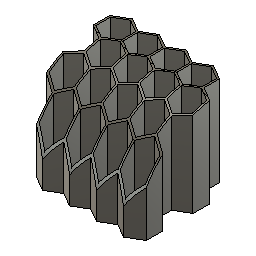
hexagon-03 (Autodesk Fusion 360 design; units mm, degrees)
Autodesk Fusion 360 part; units mm, degrees
sketch "Sketch1" plane through (0, 0, 0) normal (0, 1, 0) x (1, 0, 0)
  line L0 (16, 9.2376) -> (0, 18.4752)
  line L1 (0, 18.4752) -> (-16, 9.2376)
  line L2 (-16, 9.2376) -> (-16, -9.2376)
  line L3 (-16, -9.2376) -> (0, -18.4752)
  line L4 (0, -18.4752) -> (16, -9.2376)
  line L5 (16, -9.2376) -> (16, 9.2376)
  line L6 (46, 9.2376) -> (30, 18.4752)
  line L7 (30, 18.4752) -> (14, 9.2376)
  line L8 (14, 9.2376) -> (14, -9.2376)
  line L9 (14, -9.2376) -> (30, -18.4752)
  line L10 (30, -18.4752) -> (46, -9.2376)
  line L11 (46, -9.2376) -> (46, 9.2376)
  line L12 (14, 8.0829) -> (0, 16.1658)
  line L13 (0, 16.1658) -> (-14, 8.0829)
  line L14 (-14, 8.0829) -> (-14, -8.0829)
  line L15 (-14, -8.0829) -> (0, -16.1658)
  line L16 (0, -16.1658) -> (14, -8.0829)
  line L17 (14, -8.0829) -> (14, 8.0829)
  line L18 (44, 8.0829) -> (30, 16.1658)
  line L19 (30, 16.1658) -> (16, 8.0829)
  line L20 (16, 8.0829) -> (16, -8.0829)
  line L21 (16, -8.0829) -> (30, -16.1658)
  line L22 (30, -16.1658) -> (44, -8.0829)
  line L23 (44, -8.0829) -> (44, 8.0829)
  line L24 (15, -9.8342) -> (1, -17.9171)
  line L25 (59, -17.9171) -> (45, -9.8342)
  line L26 (15, -42.1658) -> (29, -34.0829)
  line L27 (29, -16.7624) -> (29, -35.2376)
  line L28 (-1, -16.7624) -> (-1, -35.2376)
  line L29 (29, -35.2376) -> (45, -44.4752)
  line L30 (29, -17.9171) -> (15, -9.8342)
  line L31 (61, -16.7624) -> (45, -7.5248)
  line L32 (45, -42.1658) -> (59, -34.0829)
  line L33 (59, -34.0829) -> (59, -17.9171)
  line L34 (61, -35.2376) -> (61, -16.7624)
  line L35 (45, -9.8342) -> (31, -17.9171)
  line L36 (31, -34.0829) -> (45, -42.1658)
  line L37 (15, -7.5248) -> (-1, -16.7624)
  line L38 (45, -7.5248) -> (29, -16.7624)
  line L39 (-1, -35.2376) -> (15, -44.4752)
  line L40 (45, -44.4752) -> (61, -35.2376)
  line L41 (1, -17.9171) -> (1, -34.0829)
  line L42 (31, -17.9171) -> (31, -34.0829)
  line L43 (31, -16.7624) -> (15, -7.5248)
  line L44 (15, -44.4752) -> (31, -35.2376)
  line L45 (29, -34.0829) -> (29, -17.9171)
  line L46 (1, -34.0829) -> (15, -42.1658)
  line L47 (31, -35.2376) -> (31, -16.7624)
  line L48 (89, -34.0829) -> (89, -17.9171)
  line L49 (60, -18.4752) -> (76, -9.2376)
  line L50 (76, 9.2376) -> (60, 18.4752)
  line L51 (59, -35.2376) -> (75, -44.4752)
  line L52 (75, -9.8342) -> (61, -17.9171)
  line L53 (75, -44.4752) -> (91, -35.2376)
  line L54 (75, -42.1658) -> (89, -34.0829)
  line L55 (119, -34.0829) -> (119, -17.9171)
  line L56 (121, -16.7624) -> (105, -7.5248)
  line L57 (90, -16.1658) -> (104, -8.0829)
  line L58 (105, -9.8342) -> (91, -17.9171)
  line L59 (60, 16.1658) -> (46, 8.0829)
  line L60 (44, -9.2376) -> (60, -18.4752)
  line L61 (74, -8.0829) -> (74, 8.0829)
  line L62 (74, -9.2376) -> (90, -18.4752)
  line L63 (105, -44.4752) -> (121, -35.2376)
  line L64 (74, 9.2376) -> (74, -9.2376)
  line L65 (46, 8.0829) -> (46, -8.0829)
  line L66 (59, -16.7624) -> (59, -35.2376)
  line L67 (90, 18.4752) -> (74, 9.2376)
  line L68 (76, 8.0829) -> (76, -8.0829)
  line L69 (91, -34.0829) -> (105, -42.1658)
  line L70 (89, -17.9171) -> (75, -9.8342)
  line L71 (105, -7.5248) -> (89, -16.7624)
  line L72 (119, -17.9171) -> (105, -9.8342)
  line L73 (104, 8.0829) -> (90, 16.1658)
  line L74 (60, 18.4752) -> (44, 9.2376)
  line L75 (90, 16.1658) -> (76, 8.0829)
  line L76 (90, -18.4752) -> (106, -9.2376)
  line L77 (76, -9.2376) -> (76, 9.2376)
  line L78 (106, -9.2376) -> (106, 9.2376)
  line L79 (106, 9.2376) -> (90, 18.4752)
  line L80 (74, 8.0829) -> (60, 16.1658)
  line L81 (89, -16.7624) -> (89, -35.2376)
  line L82 (61, -17.9171) -> (61, -34.0829)
  line L83 (105, -42.1658) -> (119, -34.0829)
  line L84 (91, -16.7624) -> (75, -7.5248)
  line L85 (91, -17.9171) -> (91, -34.0829)
  line L86 (91, -35.2376) -> (91, -16.7624)
  line L87 (75, -7.5248) -> (59, -16.7624)
  line L88 (121, -35.2376) -> (121, -16.7624)
  line L89 (61, -34.0829) -> (75, -42.1658)
  line L90 (76, -8.0829) -> (90, -16.1658)
  line L91 (89, -35.2376) -> (105, -44.4752)
  line L92 (46, -8.0829) -> (60, -16.1658)
  line L93 (104, -8.0829) -> (104, 8.0829)
  line L94 (44, 9.2376) -> (44, -9.2376)
  line L95 (60, -16.1658) -> (74, -8.0829)
  line L96 (16, 9.2376) -> (0, 18.4752)
  line L97 (0, -18.4752) -> (16, -9.2376)
  line L98 (0, -16.1658) -> (14, -8.0829)
  line L99 (104, -8.0829) -> (104, 8.0829)
  line L100 (90, -18.4752) -> (106, -9.2376)
  line L101 (44, 9.2376) -> (44, -9.2376)
  line L102 (-16, -9.2376) -> (0, -18.4752)
  line L103 (60, -18.4752) -> (76, -9.2376)
  line L104 (-14, 8.0829) -> (-14, -8.0829)
  line L105 (0, 16.1658) -> (-14, 8.0829)
  line L106 (90, 18.4752) -> (74, 9.2376)
  line L107 (60, 18.4752) -> (44, 9.2376)
  line L108 (76, -8.0829) -> (90, -16.1658)
  line L109 (-14, -8.0829) -> (0, -16.1658)
  line L110 (90, -16.1658) -> (104, -8.0829)
  line L111 (-1, -16.7624) -> (-1, -35.2376)
  line L112 (0, 18.4752) -> (-16, 9.2376)
  line L113 (60, -16.1658) -> (74, -8.0829)
  line L114 (1, -17.9171) -> (1, -34.0829)
  line L115 (46, -9.2376) -> (46, 9.2376)
  line L116 (44, -8.0829) -> (44, 8.0829)
  line L117 (45, -9.8342) -> (31, -17.9171)
  line L118 (30, 18.4752) -> (14, 9.2376)
  line L119 (30, -16.1658) -> (44, -8.0829)
  line L120 (59, -34.0829) -> (59, -17.9171)
  line L121 (45, -42.1658) -> (59, -34.0829)
  line L122 (89, -35.2376) -> (105, -44.4752)
  line L123 (59, -17.9171) -> (45, -9.8342)
  line L124 (31, -35.2376) -> (31, -16.7624)
  line L125 (15, -42.1658) -> (29, -34.0829)
  line L126 (14, -8.0829) -> (14, 8.0829)
  line L127 (61, -35.2376) -> (61, -16.7624)
  line L128 (31, -16.7624) -> (15, -7.5248)
  line L129 (30, 16.1658) -> (16, 8.0829)
  line L130 (61, -16.7624) -> (45, -7.5248)
  line L131 (16, -8.0829) -> (30, -16.1658)
  line L132 (15, -44.4752) -> (31, -35.2376)
  line L133 (44, 8.0829) -> (30, 16.1658)
  line L134 (61, -17.9171) -> (61, -34.0829)
  line L135 (45, -44.4752) -> (61, -35.2376)
  line L136 (60, 16.1658) -> (46, 8.0829)
  line L137 (16, -9.2376) -> (16, 9.2376)
  line L138 (14, 9.2376) -> (14, -9.2376)
  line L139 (45, -7.5248) -> (29, -16.7624)
  line L140 (29, -16.7624) -> (29, -35.2376)
  line L141 (30, -18.4752) -> (46, -9.2376)
  line L142 (14, -9.2376) -> (30, -18.4752)
  line L143 (14, 8.0829) -> (0, 16.1658)
  line L144 (1, -34.0829) -> (15, -42.1658)
  line L145 (15, -7.5248) -> (-1, -16.7624)
  line L146 (-1, -35.2376) -> (15, -44.4752)
  line L147 (121, -35.2376) -> (121, -16.7624)
  line L148 (31, -17.9171) -> (31, -34.0829)
  line L149 (105, -42.1658) -> (119, -34.0829)
  line L150 (91, -35.2376) -> (91, -16.7624)
  line L151 (119, -34.0829) -> (119, -17.9171)
  line L152 (91, -34.0829) -> (105, -42.1658)
  line L153 (59, -16.7624) -> (59, -35.2376)
  line L154 (31, -34.0829) -> (45, -42.1658)
  line L155 (29, -34.0829) -> (29, -17.9171)
  line L156 (29, -35.2376) -> (45, -44.4752)
  line L157 (75, -44.4752) -> (91, -35.2376)
  line L158 (89, -34.0829) -> (89, -17.9171)
  line L159 (75, -42.1658) -> (89, -34.0829)
  line L160 (59, -35.2376) -> (75, -44.4752)
  line L161 (16, 8.0829) -> (16, -8.0829)
  line L162 (29, -17.9171) -> (15, -9.8342)
  line L163 (89, -16.7624) -> (89, -35.2376)
  line L164 (105, -44.4752) -> (121, -35.2376)
  line L165 (91, -17.9171) -> (91, -34.0829)
  line L166 (61, -34.0829) -> (75, -42.1658)
  line L167 (106, 9.2376) -> (90, 18.4752)
  line L168 (15, -9.8342) -> (1, -17.9171)
  line L169 (-16, 9.2376) -> (-16, -9.2376)
  line L170 (74, -8.0829) -> (74, 8.0829)
  line L171 (90, 16.1658) -> (76, 8.0829)
  line L172 (76, 8.0829) -> (76, -8.0829)
  line L173 (75, -9.8342) -> (61, -17.9171)
  line L174 (121, -16.7624) -> (105, -7.5248)
  line L175 (106, -9.2376) -> (106, 9.2376)
  line L176 (76, 9.2376) -> (60, 18.4752)
  line L177 (91, -16.7624) -> (75, -7.5248)
  line L178 (105, -9.8342) -> (91, -17.9171)
  line L179 (46, 8.0829) -> (46, -8.0829)
  line L180 (105, -7.5248) -> (89, -16.7624)
  line L181 (46, 9.2376) -> (30, 18.4752)
  line L182 (89, -17.9171) -> (75, -9.8342)
  line L183 (46, -8.0829) -> (60, -16.1658)
  line L184 (104, 8.0829) -> (90, 16.1658)
  line L185 (76, -9.2376) -> (76, 9.2376)
  line L186 (119, -17.9171) -> (105, -9.8342)
  line L187 (74, 8.0829) -> (60, 16.1658)
  line L188 (74, -9.2376) -> (90, -18.4752)
  line L189 (44, -9.2376) -> (60, -18.4752)
  line L190 (75, -7.5248) -> (59, -16.7624)
  line L191 (74, 9.2376) -> (74, -9.2376)
  line L192 (15, -59.5248) -> (-1, -68.7624)
  line L193 (59, -68.7624) -> (59, -87.2376)
  line L194 (91, -69.9171) -> (91, -86.0829)
  line L195 (105, -94.1658) -> (119, -86.0829)
  line L196 (31, -87.2376) -> (31, -68.7624)
  line L197 (31, -69.9171) -> (31, -86.0829)
  line L198 (15, -96.4752) -> (31, -87.2376)
  line L199 (121, -87.2376) -> (121, -68.7624)
  line L200 (45, -96.4752) -> (61, -87.2376)
  line L201 (119, -86.0829) -> (119, -69.9171)
  line L202 (31, -86.0829) -> (45, -94.1658)
  line L203 (89, -86.0829) -> (89, -69.9171)
  line L204 (29, -87.2376) -> (45, -96.4752)
  line L205 (89, -86.0829) -> (89, -69.9171)
  line L206 (89, -87.2376) -> (105, -96.4752)
  line L207 (89, -87.2376) -> (105, -96.4752)
  line L208 (89, -68.7624) -> (89, -87.2376)
  line L209 (61, -69.9171) -> (61, -86.0829)
  line L210 (91, -86.0829) -> (105, -94.1658)
  line L211 (105, -96.4752) -> (121, -87.2376)
  line L212 (91, -87.2376) -> (91, -68.7624)
  line L213 (91, -86.0829) -> (105, -94.1658)
  line L214 (61, -87.2376) -> (61, -68.7624)
  line L215 (45, -94.1658) -> (59, -86.0829)
  line L216 (75, -96.4752) -> (91, -87.2376)
  line L217 (75, -94.1658) -> (89, -86.0829)
  line L218 (15, -94.1658) -> (29, -86.0829)
  line L219 (29, -86.0829) -> (29, -69.9171)
  line L220 (1, -86.0829) -> (15, -94.1658)
  line L221 (74, -42.7624) -> (74, -61.2376)
  line L222 (74, -60.0829) -> (74, -43.9171)
  line L223 (15, -61.8342) -> (1, -69.9171)
  line L224 (-1, -87.2376) -> (15, -96.4752)
  line L225 (14, -43.9171) -> (0, -35.8342)
  line L226 (0, -70.4752) -> (16, -61.2376)
  line L227 (104, -60.0829) -> (104, -43.9171)
  line L228 (44, -60.0829) -> (44, -43.9171)
  line L229 (0, -68.1658) -> (14, -60.0829)
  line L230 (106, -42.7624) -> (90, -33.5248)
  line L231 (0, -68.1658) -> (14, -60.0829)
  line L232 (90, -35.8342) -> (76, -43.9171)
  line L233 (46, -43.9171) -> (46, -60.0829)
  line L234 (14, -43.9171) -> (0, -35.8342)
  line L235 (106, -61.2376) -> (106, -42.7624)
  line L236 (90, -33.5248) -> (74, -42.7624)
  line L237 (16, -42.7624) -> (0, -33.5248)
  line L238 (-1, -87.2376) -> (15, -96.4752)
  line L239 (76, -42.7624) -> (60, -33.5248)
  line L240 (-14, -60.0829) -> (0, -68.1658)
  line L241 (-1, -68.7624) -> (-1, -87.2376)
  line L242 (0, -35.8342) -> (-14, -43.9171)
  line L243 (74, -61.2376) -> (90, -70.4752)
  line L244 (15, -59.5248) -> (-1, -68.7624)
  line L245 (0, -70.4752) -> (16, -61.2376)
  line L246 (76, -61.2376) -> (76, -42.7624)
  line L247 (-1, -68.7624) -> (-1, -87.2376)
  line L248 (44, -42.7624) -> (44, -61.2376)
  line L249 (-16, -42.7624) -> (-16, -61.2376)
  line L250 (75, -59.5248) -> (59, -68.7624)
  line L251 (74, -43.9171) -> (60, -35.8342)
  line L252 (1, -86.0829) -> (15, -94.1658)
  line L253 (60, -35.8342) -> (46, -43.9171)
  line L254 (1, -69.9171) -> (1, -86.0829)
  line L255 (104, -43.9171) -> (90, -35.8342)
  line L256 (46, -60.0829) -> (60, -68.1658)
  line L257 (15, -61.8342) -> (1, -69.9171)
  line L258 (-14, -43.9171) -> (-14, -60.0829)
  line L259 (30, -68.1658) -> (44, -60.0829)
  line L260 (-16, -61.2376) -> (0, -70.4752)
  line L261 (-14, -60.0829) -> (0, -68.1658)
  line L262 (45, -59.5248) -> (29, -68.7624)
  line L263 (46, -61.2376) -> (46, -42.7624)
  line L264 (-16, -61.2376) -> (0, -70.4752)
  line L265 (16, -42.7624) -> (0, -33.5248)
  line L266 (0, -33.5248) -> (-16, -42.7624)
  line L267 (60, -33.5248) -> (44, -42.7624)
  line L268 (14, -61.2376) -> (30, -70.4752)
  line L269 (1, -69.9171) -> (1, -86.0829)
  line L270 (-14, -43.9171) -> (-14, -60.0829)
  line L271 (0, -35.8342) -> (-14, -43.9171)
  line L272 (44, -61.2376) -> (60, -70.4752)
  line L273 (45, -96.4752) -> (61, -87.2376)
  line L274 (89, -68.7624) -> (89, -87.2376)
  line L275 (29, -86.0829) -> (29, -69.9171)
  line L276 (60, -70.4752) -> (76, -61.2376)
  line L277 (46, -60.0829) -> (60, -68.1658)
  line L278 (30, -35.8342) -> (16, -43.9171)
  line L279 (16, -60.0829) -> (30, -68.1658)
  line L280 (30, -33.5248) -> (14, -42.7624)
  line L281 (44, -43.9171) -> (30, -35.8342)
  line L282 (59, -87.2376) -> (75, -96.4752)
  line L283 (59, -68.7624) -> (59, -87.2376)
  line L284 (60, -68.1658) -> (74, -60.0829)
  line L285 (14, -61.2376) -> (30, -70.4752)
  line L286 (105, -96.4752) -> (121, -87.2376)
  line L287 (44, -43.9171) -> (30, -35.8342)
  line L288 (30, -33.5248) -> (14, -42.7624)
  line L289 (31, -69.9171) -> (31, -86.0829)
  line L290 (29, -87.2376) -> (45, -96.4752)
  line L291 (31, -86.0829) -> (45, -94.1658)
  line L292 (59, -86.0829) -> (59, -69.9171)
  line L293 (121, -68.7624) -> (105, -59.5248)
  line L294 (61, -68.7624) -> (45, -59.5248)
  line L295 (90, -68.1658) -> (104, -60.0829)
  line L296 (45, -59.5248) -> (29, -68.7624)
  line L297 (89, -69.9171) -> (75, -61.8342)
  line L298 (59, -69.9171) -> (45, -61.8342)
  line L299 (15, -94.1658) -> (29, -86.0829)
  line L300 (91, -87.2376) -> (91, -68.7624)
  line L301 (15, -96.4752) -> (31, -87.2376)
  line L302 (61, -69.9171) -> (61, -86.0829)
  line L303 (105, -94.1658) -> (119, -86.0829)
  line L304 (75, -94.1658) -> (89, -86.0829)
  line L305 (29, -69.9171) -> (15, -61.8342)
  line L306 (75, -59.5248) -> (59, -68.7624)
  line L307 (45, -61.8342) -> (31, -69.9171)
  line L308 (30, -35.8342) -> (16, -43.9171)
  line L309 (14, -42.7624) -> (14, -61.2376)
  line L310 (30, -68.1658) -> (44, -60.0829)
  line L311 (74, -61.2376) -> (90, -70.4752)
  line L312 (16, -43.9171) -> (16, -60.0829)
  line L313 (105, -59.5248) -> (89, -68.7624)
  line L314 (61, -86.0829) -> (75, -94.1658)
  line L315 (61, -86.0829) -> (75, -94.1658)
  line L316 (119, -69.9171) -> (105, -61.8342)
  line L317 (119, -86.0829) -> (119, -69.9171)
  line L318 (91, -68.7624) -> (75, -59.5248)
  line L319 (31, -87.2376) -> (31, -68.7624)
  line L320 (121, -87.2376) -> (121, -68.7624)
  line L321 (30, -70.4752) -> (46, -61.2376)
  line L322 (76, -60.0829) -> (90, -68.1658)
  line L323 (31, -68.7624) -> (15, -59.5248)
  line L324 (46, -42.7624) -> (30, -33.5248)
  line L325 (59, -87.2376) -> (75, -96.4752)
  line L326 (46, -42.7624) -> (30, -33.5248)
  line L327 (61, -87.2376) -> (61, -68.7624)
  line L328 (45, -94.1658) -> (59, -86.0829)
  line L329 (105, -61.8342) -> (91, -69.9171)
  line L330 (75, -61.8342) -> (61, -69.9171)
  line L331 (59, -86.0829) -> (59, -69.9171)
  line L332 (29, -68.7624) -> (29, -87.2376)
  line L333 (91, -69.9171) -> (91, -86.0829)
  line L334 (29, -68.7624) -> (29, -87.2376)
  line L335 (75, -96.4752) -> (91, -87.2376)
  line L336 (74, -60.0829) -> (74, -43.9171)
  line L337 (76, -43.9171) -> (76, -60.0829)
  line L338 (46, -61.2376) -> (46, -42.7624)
  line L339 (60, -33.5248) -> (44, -42.7624)
  line L340 (44, -60.0829) -> (44, -43.9171)
  line L341 (60, -35.8342) -> (46, -43.9171)
  line L342 (74, -42.7624) -> (74, -61.2376)
  line L343 (91, -68.7624) -> (75, -59.5248)
  line L344 (121, -68.7624) -> (105, -59.5248)
  line L345 (0, -33.5248) -> (-16, -42.7624)
  line L346 (90, -33.5248) -> (74, -42.7624)
  line L347 (105, -59.5248) -> (89, -68.7624)
  line L348 (60, -70.4752) -> (76, -61.2376)
  line L349 (119, -69.9171) -> (105, -61.8342)
  line L350 (31, -68.7624) -> (15, -59.5248)
  line L351 (90, -70.4752) -> (106, -61.2376)
  line L352 (104, -60.0829) -> (104, -43.9171)
  line L353 (90, -70.4752) -> (106, -61.2376)
  line L354 (76, -42.7624) -> (60, -33.5248)
  line L355 (-16, -42.7624) -> (-16, -61.2376)
  line L356 (16, -43.9171) -> (16, -60.0829)
  line L357 (90, -35.8342) -> (76, -43.9171)
  line L358 (14, -60.0829) -> (14, -43.9171)
  line L359 (105, -61.8342) -> (91, -69.9171)
  line L360 (16, -61.2376) -> (16, -42.7624)
  line L361 (45, -61.8342) -> (31, -69.9171)
  line L362 (44, -42.7624) -> (44, -61.2376)
  line L363 (90, -68.1658) -> (104, -60.0829)
  line L364 (30, -70.4752) -> (46, -61.2376)
  line L365 (76, -61.2376) -> (76, -42.7624)
  line L366 (89, -69.9171) -> (75, -61.8342)
  line L367 (60, -68.1658) -> (74, -60.0829)
  line L368 (59, -69.9171) -> (45, -61.8342)
  line L369 (16, -61.2376) -> (16, -42.7624)
  line L370 (29, -69.9171) -> (15, -61.8342)
  line L371 (16, -60.0829) -> (30, -68.1658)
  line L372 (61, -68.7624) -> (45, -59.5248)
  line L373 (44, -61.2376) -> (60, -70.4752)
  line L374 (74, -43.9171) -> (60, -35.8342)
  line L375 (106, -61.2376) -> (106, -42.7624)
  line L376 (76, -60.0829) -> (90, -68.1658)
  line L377 (104, -43.9171) -> (90, -35.8342)
  line L378 (46, -43.9171) -> (46, -60.0829)
  line L379 (14, -42.7624) -> (14, -61.2376)
  line L380 (106, -42.7624) -> (90, -33.5248)
  line L381 (14, -60.0829) -> (14, -43.9171)
  line L382 (75, -61.8342) -> (61, -69.9171)
  line L383 (76, -43.9171) -> (76, -60.0829)
  point P0 (30, 0)
  point P1 (30, 0)
  point P2 (15, -26)
  point P3 (15, -26)
  point P4 (45, -26)
  point P5 (15, -26)
  point P6 (45, -26)
  point P7 (75, -26)
  point P8 (75, -26)
  point P9 (105, -26)
  point P10 (75, -26)
  point P11 (105, -26)
  point P12 (60, 0)
  point P13 (60, 0)
  point P14 (90, 0)
  point P15 (60, 0)
  point P16 (90, 0)
  point P17 (15, -26)
  point P18 (15, -26)
  point P19 (45, -26)
  point P20 (15, -26)
  point P21 (45, -26)
  point P22 (105, -26)
  point P23 (60, 0)
  point P24 (105, -26)
  point P25 (90, 0)
  point P26 (90, 0)
  point P27 (60, 0)
  point P28 (75, -26)
  point P29 (75, -26)
  point P30 (75, -26)
  point P31 (60, 0)
  point P32 (30, 0)
  point P33 (30, 0)
  point P34 (60, -52)
  point P35 (75, -78)
  point P36 (60, -52)
  point P37 (90, -52)
  point P38 (90, -52)
  point P39 (75, -78)
  point P40 (60, -52)
  point P41 (0, -52)
  point P42 (105, -78)
  point P43 (30, -52)
  point P44 (75, -78)
  point P45 (0, -52)
  point P46 (105, -78)
  point P47 (0, -52)
  point P48 (15, -78)
  point P49 (45, -78)
  point P50 (15, -78)
  point P51 (15, -78)
  point P52 (45, -78)
  point P53 (15, -78)
  point P54 (15, -78)
  point P55 (45, -78)
  point P56 (15, -78)
  point P57 (45, -78)
  point P58 (105, -78)
  point P59 (60, -52)
  point P60 (105, -78)
  point P61 (90, -52)
  point P62 (90, -52)
  point P63 (60, -52)
  point P64 (75, -78)
  point P65 (75, -78)
  point P66 (75, -78)
  point P67 (60, -52)
  point P68 (0, -52)
  point P69 (0, -52)
  point P70 (30, -52)
  point P71 (30, -52)
  point P72 (0, -52)
  point P73 (30, -52)
  dimension "d7" = 16
  dimension "d8" = 16
  dimension "d9" = 2
  dimension "d10" = 14
  dimension "d11" = 14
  dimension "d14" = 16
  dimension "d15" = 16
  dimension "d16" = 2
  dimension "d17" = 14
  dimension "d18" = 14
  dimension "d19" = 16
  dimension "d20" = 16
  dimension "d21" = 2
  dimension "d22" = 14
  dimension "d23" = 14
  dimension "d24" = 16
  dimension "d25" = 16
  dimension "d26" = 2
  dimension "d27" = 14
  dimension "d28" = 14
  dimension "d29" = 16
  dimension "d30" = 16
  dimension "d31" = 2
  dimension "d32" = 14
  dimension "d33" = 14
  dimension "d34" = 16
  dimension "d35" = 16
  dimension "d36" = 2
  dimension "d37" = 14
  dimension "d38" = 14
  dimension "d39" = 16
  dimension "d40" = 16
  dimension "d41" = 2
  dimension "d42" = 14
  dimension "d43" = 14
  dimension "d44" = 16
  dimension "d45" = 16
  dimension "d46" = 2
  dimension "d47" = 14
  dimension "d48" = 14
  dimension "d49" = 16
  dimension "d50" = 16
  dimension "d51" = 2
  dimension "d52" = 14
  dimension "d53" = 14
  dimension "d54" = 16
  dimension "d55" = 16
  dimension "d56" = 2
  dimension "d57" = 14
  dimension "d58" = 14
  dimension "d59" = 16
  dimension "d60" = 16
  dimension "d61" = 2
  dimension "d62" = 14
  dimension "d63" = 14
  dimension "d64" = 16
  dimension "d65" = 16
  dimension "d66" = 2
  dimension "d67" = 14
  dimension "d68" = 14
  dimension "d69" = 16
  dimension "d70" = 16
  dimension "d71" = 2
  dimension "d72" = 14
  dimension "d73" = 14
  dimension "d74" = 16
  dimension "d75" = 16
  dimension "d76" = 2
  dimension "d77" = 14
  dimension "d78" = 14
  dimension "d79" = 16
  dimension "d80" = 16
  dimension "d81" = 2
  dimension "d82" = 14
  dimension "d83" = 14
  dimension "d84" = 16
  dimension "d85" = 16
  dimension "d86" = 2
  dimension "d87" = 14
  dimension "d88" = 14
  constraint coincident P33 P32
  constraint coincident P20 P18
  constraint coincident P21 P19
  constraint coincident P31 P27
  constraint coincident P26 P25
  constraint coincident P30 P29
  constraint coincident P24 P22
  constraint coincident P72 P69
  constraint coincident P73 P71
  constraint coincident P56 P54
  constraint coincident P57 P55
  constraint coincident P67 P63
  constraint coincident P62 P61
  constraint coincident P66 P65
  constraint coincident P60 P58
  measures "d7" distance of origin L5
  measures "d8" distance of P33 L11
  measures "d9" distance of L5 L8
  measures "d10" distance of origin L17
  measures "d11" distance of P33 L23
  measures "d14" distance of P20 L47
  measures "d15" distance of P21 L34
  measures "d16" distance of L27 L47
  measures "d17" distance of P20 L45
  measures "d18" distance of P21 L33
  measures "d19" distance of P31 L77
  measures "d20" distance of P26 L78
  measures "d21" distance of L64 L77
  measures "d22" distance of P31 L61
  measures "d23" distance of P26 L93
  measures "d24" distance of P30 L86
  measures "d25" distance of P24 L88
  measures "d26" distance of L81 L86
  measures "d27" distance of P30 L48
  measures "d28" distance of P24 L55
  measures "d29" distance of origin L137
  measures "d30" distance of P33 L115
  measures "d31" distance of L137 L138
  measures "d32" distance of origin L126
  measures "d33" distance of P33 L116
  measures "d34" distance of P20 L124
  measures "d35" distance of P21 L127
  measures "d36" distance of L124 L140
  measures "d37" distance of P20 L155
  measures "d38" distance of P21 L120
  measures "d39" distance of P31 L185
  measures "d40" distance of P26 L175
  measures "d41" distance of L185 L191
  measures "d42" distance of P31 L170
  measures "d43" distance of P26 L99
  measures "d44" distance of P30 L150
  measures "d45" distance of P24 L147
  measures "d46" distance of L150 L163
  measures "d47" distance of P30 L158
  measures "d48" distance of P24 L151
  measures "d49" distance of P72 L360
  measures "d50" distance of P73 L338
  measures "d51" distance of L309 L360
  measures "d52" distance of P72 L381
  measures "d53" distance of P73 L340
  measures "d54" distance of P56 L319
  measures "d55" distance of P57 L327
  measures "d56" distance of L319 L332
  measures "d57" distance of P56 L275
  measures "d58" distance of P57 L331
  measures "d59" distance of P67 L365
  measures "d60" distance of P62 L375
  measures "d61" distance of L342 L365
  measures "d62" distance of P67 L336
  measures "d63" distance of P62 L352
  measures "d64" distance of P66 L300
  measures "d65" distance of P60 L320
  measures "d66" distance of L274 L300
  measures "d67" distance of P66 L203
  measures "d68" distance of P60 L317
  measures "d69" distance of P72 L369
  measures "d70" distance of P73 L263
  measures "d71" distance of L369 L379
  measures "d72" distance of P72 L358
  measures "d73" distance of P73 L228
  measures "d74" distance of P56 L196
  measures "d75" distance of P57 L214
  measures "d76" distance of L196 L334
  measures "d77" distance of P56 L219
  measures "d78" distance of P57 L292
  measures "d79" distance of P67 L246
  measures "d80" distance of P62 L235
  measures "d81" distance of L221 L246
  measures "d82" distance of P67 L222
  measures "d83" distance of P62 L227
  measures "d84" distance of P66 L212
  measures "d85" distance of P60 L199
  measures "d86" distance of L208 L212
  measures "d87" distance of P66 L205
  measures "d88" distance of P60 L201
extrude "Extrude2" add sketch "Sketch1" along normal blind 100 contours L0 L5 L7 L8 L17 L20 L37 L43 L96 L118 L126 L128 L137 L138 L145 L161 | L0 L5 L6 L7 L18 L19 L74 L94 L96 L101 L107 L118 L129 L133 L137 L181 | L0 L1 L2 L3 L7 L8 L12 L13 L14 L15 L16 L28 L37 L96 L98 L102 L104 L105 L109 L111 L112 L118 L138 L143 L145 L169 | L5 L21 L22 L38 L43 L94 L101 L119 L128 L131 L137 L139 | L6 L11 L50 L59 L64 L67 L74 L80 L106 L107 L115 L136 L176 L181 L187 L191 | L6 L11 L23 L31 L38 L65 L74 L94 L101 L107 L115 L116 L130 L139 L179 L181 | L4 L5 L9 L27 L38 L43 L97 L128 L137 L139 L140 L142 | L4 L5 L8 L9 L37 L43 L97 L128 L137 L138 L142 L145 | L9 L10 L27 L38 L43 L47 L124 L128 L139 L140 L141 L142 | L10 L38 L43 L47 L60 L94 L101 L124 L128 L139 L141 L189 | L3 L4 L8 L9 L28 L37 L97 L102 L111 L138 L142 L145 | L3 L4 L9 L24 L26 L27 L28 L30 L41 L46 L97 L102 L111 L114 L125 L140 L142 L144 L162 L168 L237 L265 L266 L280 L288 L345 | L50 L56 L57 L67 L71 L73 L75 L77 L78 L79 L84 L90 L93 L99 L106 L108 L110 L167 L171 L174 L175 L176 L177 L180 L184 L185 | L50 L61 L64 L67 L68 L77 L84 L87 L106 L170 L172 L176 L177 L185 L190 L191 | L10 L11 L31 L38 L60 L94 L101 L115 L130 L139 L141 L189 | L28 L39 L111 L146 L237 L265 L266 L280 L288 L309 L345 L379 | L28 L39 L111 L146 L192 L225 L229 L231 L234 L240 L241 L242 L244 L247 L249 L258 L260 L261 L264 L266 L270 L271 L309 L345 L355 L379 | L11 L31 L64 L87 L92 L95 L113 L115 L130 L183 L190 L191 | L9 L10 L27 L42 L45 L47 L124 L140 L141 L142 L148 L155 L280 L288 L324 L326 | L10 L25 L35 L47 L60 L66 L117 L123 L124 L141 L153 L189 | L10 L11 L31 L60 L66 L87 L115 L130 L141 L153 L189 L190 | L39 L44 L132 L146 L237 L265 L280 L288 L309 L360 L369 L379 | L39 L44 L132 L146 L192 L244 L309 L312 L323 L350 L356 L358 L360 L369 L379 L381 | L27 L29 L44 L132 L140 L156 L237 L265 L280 L288 L360 L369 | L31 L34 L49 L62 L64 L87 L103 L127 L130 L188 L190 L191 | L31 L34 L49 L60 L66 L87 L103 L127 L130 L153 L189 L190 | L56 L71 L76 L78 L84 L86 L100 L150 L174 L175 L177 L180 | L55 L56 L58 L63 L69 L72 L76 L78 L83 L86 L88 L100 L147 L149 L150 L151 L152 L164 L174 L175 L178 L186 L230 L235 L375 L380 | L33 L34 L49 L60 L66 L82 L103 L120 L127 L134 L153 L189 L239 L267 L339 L354 | L32 L36 L47 L66 L121 L124 L153 L154 L267 L324 L326 L339 | L27 L29 L44 L47 L124 L132 L140 L156 L280 L288 L324 L326 | L198 L204 L218 L220 L223 L224 L226 L238 L241 L245 L247 L252 L254 L257 L260 L264 L268 L269 L285 L290 L299 L301 L305 L332 L334 L370 | L192 L226 L241 L244 L245 L247 L260 L264 L268 L285 L309 L379 | L49 L62 L64 L77 L84 L87 L103 L177 L185 L188 L190 L191 | L49 L62 L71 L77 L81 L84 L103 L163 L177 L180 L185 L188 | L29 L44 L47 L124 L132 L156 L248 L267 L324 L326 L339 L362 | L29 L44 L132 L156 L248 L278 L281 L287 L308 L360 L362 L369 | L34 L49 L52 L62 L70 L81 L103 L127 L163 L173 L182 L188 | L62 L71 L76 L81 L84 L86 L100 L150 L163 L177 L180 L188 | L48 L62 L76 L81 L85 L86 L100 L150 L158 L163 L165 L188 L230 L236 L346 L380 | L29 L40 L135 L156 L248 L263 L267 L324 L326 L338 L339 L362 | L40 L51 L66 L135 L153 L160 L263 L267 L324 L326 L338 L339 | L192 L226 L244 L245 L268 L285 L309 L323 L350 L360 L369 L379 | L226 L245 L262 L268 L285 L296 L323 L332 L334 L350 L360 L369 | L53 L63 L91 L122 L157 L164 L227 L232 L235 L246 L255 L293 L295 L313 L318 L322 L343 L344 L347 L352 L357 L363 L365 L375 L376 L377 | L53 L63 L86 L91 L122 L150 L157 L164 L230 L235 L375 L380 | L34 L40 L51 L66 L127 L135 L153 L160 L239 L267 L339 L354 | L29 L40 L135 L156 L228 L233 L248 L262 L263 L294 L296 L338 L340 L362 L372 L378 | L248 L259 L262 L279 L296 L310 L323 L350 L360 L362 L369 L371 | L196 L197 L198 L204 L219 L268 L275 L285 L289 L290 L301 L319 L321 L332 L334 L364 | L193 L196 L198 L200 L202 L204 L215 L273 L282 L283 L290 L291 L301 L319 L325 L328 | L196 L262 L268 L285 L296 L319 L321 L323 L332 L334 L350 L364 | L34 L54 L81 L89 L127 L159 L163 L166 L236 L239 L346 L354 | L195 L199 L201 L206 L207 L210 L211 L212 L213 L216 L235 L286 L293 L300 L303 L316 L317 L320 L329 L335 L344 L349 L351 L353 L359 L375 | L212 L235 L293 L300 L313 L318 L343 L344 L347 L351 L353 L375 | L40 L51 L135 L160 L221 L251 L253 L263 L338 L341 L342 L374 | L34 L40 L51 L127 L135 L160 L221 L236 L239 L342 L346 L354 | L53 L81 L86 L91 L122 L150 L157 L163 L230 L236 L346 L380 | L53 L81 L91 L122 L157 L163 L236 L239 L246 L346 L354 L365 | L196 L248 L262 L272 L296 L319 L321 L323 L350 L362 L364 L373 | L193 L200 L209 L214 L272 L273 L276 L282 L283 L292 L302 L325 L327 L331 L348 L373 | L200 L206 L207 L208 L214 L216 L217 L273 L274 L282 L304 L314 L315 L325 L327 L335 | L193 L196 L272 L283 L298 L307 L319 L321 L361 L364 L368 L373 | L51 L53 L157 L160 L221 L236 L239 L246 L342 L346 L354 L365 | L51 L53 L157 L160 L221 L222 L246 L250 L306 L318 L336 L337 L342 L343 L365 L383 | L208 L212 L243 L274 L300 L311 L313 L318 L343 L347 L351 L353 | L194 L203 L205 L206 L207 L208 L212 L216 L243 L274 L300 L311 L333 L335 L351 L353 | L208 L243 L246 L274 L276 L311 L313 L318 L343 L347 L348 L365 | L221 L250 L256 L263 L277 L284 L294 L306 L338 L342 L367 L372 | L248 L262 L263 L272 L294 L296 L321 L338 L362 L364 L372 L373 | L193 L250 L263 L272 L283 L294 L306 L321 L338 L364 L372 L373 | L221 L243 L246 L250 L276 L306 L311 L318 L342 L343 L348 L365 | L193 L214 L250 L272 L276 L283 L294 L306 L327 L348 L372 L373 | L208 L214 L243 L274 L276 L297 L311 L327 L330 L348 L366 L382 | L214 L221 L243 L250 L276 L294 L306 L311 L327 L342 L348 L372
extrude "Extrude3" add sketch "Sketch1" along normal blind 3
sketch "Sketch2" plane through (0, 0, 0) normal (1, 0, 0) x (0, 0, -1)
  circle A0 centre (0, 0) radius 100.9277
  line L0 (0, 100.9277) -> (-120.0555, 100.9277)
  line L1 (-100.9261, -0.5759) -> (-100.9261, 117.8677)
  constraint coincident A0.centre origin
  constraint coincident A0 L0.start
  constraint tangent A0 L0
  constraint horizontal L0
  constraint coincident A0 L1.start
  constraint perpendicular L0 L1
extrude "Extrude4" cut sketch "Sketch2" along normal blind 169 and the other way blind 53 contours A0 L0 L1
sketch "Sketch3" plane through (0, 0, 0) normal (0, 1, 0) x (1, 0, 0)
  circle A0 centre (0, 0) radius 1.5
  circle A1 centre (30, 0) radius 1.5
  circle A2 centre (15, -26) radius 1.5
  circle A3 centre (0, -52) radius 1.5
  circle A4 centre (15, -78) radius 1.5
  circle A5 centre (45, -78) radius 1.5
  circle A6 centre (30, -52) radius 1.5
  circle A7 centre (45, -26) radius 1.5
  circle A8 centre (60, 0) radius 1.5
  circle A9 centre (90, 0) radius 1.5
  circle A10 centre (105, -26) radius 1.5
  circle A11 centre (75, -26) radius 1.5
  circle A12 centre (60, -52) radius 1.5
  circle A13 centre (75, -78) radius 1.5
  circle A14 centre (105, -78) radius 1.5
  circle A15 centre (90, -52) radius 1.5
  point P0 (15, -78)
  point P1 (0, -52)
  point P2 (30, -52)
  point P3 (15, -26)
  point P4 (30, 0)
  point P5 (45, -26)
  point P6 (60, 0)
  point P7 (90, 0)
  point P8 (75, -26)
  point P9 (105, -26)
  point P10 (90, -52)
  point P11 (60, -52)
  point P12 (45, -78)
  point P13 (75, -78)
  point P14 (105, -78)
  dimension "d97" = 3
  constraint coincident A0.centre origin
  constraint coincident P4 A1.centre
  constraint coincident P3 A2.centre
  constraint coincident P1 A3.centre
  constraint coincident P0 A4.centre
  constraint coincident P12 A5.centre
  constraint coincident P2 A6.centre
  constraint coincident P5 A7.centre
  constraint coincident P6 A8.centre
  constraint coincident P7 A9.centre
  constraint coincident P9 A10.centre
  constraint coincident P8 A11.centre
  constraint coincident P11 A12.centre
  constraint coincident P13 A13.centre
  constraint coincident P14 A14.centre
  constraint coincident P10 A15.centre
  constraint equal A4 A5
  constraint equal A5 A13
  constraint equal A13 A14
  constraint equal A3 A14
  constraint equal A3 A6
  constraint equal A6 A12
  constraint equal A12 A15
  constraint equal A2 A15
  constraint equal A2 A7
  constraint equal A7 A11
  constraint equal A10 A11
  constraint equal A0 A10
  constraint equal A0 A1
  constraint equal A1 A8
  constraint equal A8 A9
  measures "d97" diameter of A0
